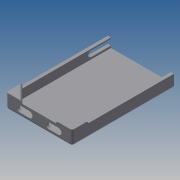
# Autodesk Inventor part: Attempt 3
Saved by Autodesk Inventor 2014 (Build 180170000, 170)
## iProperties
Created: 2014-04-30
Part Number: Attempt 3
Material: Generic
Document SubType Name: Modeling
Designer: 1770749
Density: 1 g/cm^3
Appearance: Default
Author: 1770749
Autodesk Inventor part; units mm, degrees
ref_plane "YZ Plane" through (0, 0, 0) normal (1, 0, 0) x (0, 1, 0)
ref_plane "XZ Plane" through (0, 0, 0) normal (0, 1, 0) x (-1, 0, 0)
ref_plane "XY Plane" through (0, 0, 0) normal (0, 0, 1) x (1, 0, 0)
sketch "Sketch1" plane through (0, 0, 0) normal (0, 0, 1) x (1, 0, 0)
  line L0 (0, 0) -> (59.18, 0)
  line L1 (59.18, 0) -> (59.18, 124.44)
  line L2 (59.18, 124.44) -> (0, 124.44)
  line L3 (0, 124.44) -> (0, 0)
  dimension "d0" = 59.18
  dimension "d1" = 124.44
  constraints: 8 end point, 2 parallel, 1 horizontal, 1 perpendicular
  measures "d0" distance of L2.end L1.end
  measures "d1" distance of L1.end L0.end
sketch "Sketch2" plane through (0, 0, 0) normal (0, 0, 1) x (1, 0, 0)
  line L0 (-3, 127.44) -> (62.18, 127.44)
  line L1 (62.18, 127.44) -> (62.18, -3)
  line L2 (62.18, -3) -> (-3, -3)
  line L3 (-3, -3) -> (-3, 127.44)
  line L4 (59.18, 0) -> (59.18, 124.44) projected
  line L5 (59.18, 124.44) -> (0, 124.44) projected
  line L6 (0, 124.44) -> (0, 0) projected
  line L7 (0, 0) -> (59.18, 0) projected
  dimension "d2" = 3
  dimension "d3" = 3
  dimension "d4" = 3
  dimension "d5" = 3
  constraints: 8 end point, 2 parallel, 1 horizontal, 1 perpendicular
  measures "d2" distance between parallel lines of L1 L4
  measures "d3" distance between parallel lines of L0 L5
  measures "d4" distance between parallel lines of L6 L3
  measures "d5" distance between parallel lines of L2 L7
extrude "Main Extrusion" add sketch "Sketch2" against normal blind 12 contours L0 L1 L2 L3 | L7 L6 L5 L4
extrude "Space for phone" cut sketch "Sketch1" against normal blind 8.97
fillet "Top right corner" radius 2 1 edges at (62.18, 127.44, -6)
fillet "Top left corver" radius 2 1 edges at (-3, 127.44, -6)
fillet "Botton corners" radius 2 2 edges at (62.18, -3, -6) (-3, -3, -6)
fillet "Fillet4" radius 2 8 edges at (61.5942, -2.4142, -12) (29.59, -3, -12) (-2.4142, -2.4142, -12) (-3, 62.22, -12) (-2.4142, 126.8542, -12) (29.59, 127.44, -12) (61.5942, 126.8542, -12) (62.18, 62.22, -12)
sketch "Sketch5" plane through (0, 0, 0) normal (0, 0, 1) x (1, 0, 0)
  arc A0 (-3, -1) -> (-1, -3) centre (-1, -1) ccw projected
  line L0 (60.18, -3) -> (-1, -3) projected
  line L1 (-3, -1) -> (-3, 125.44) projected
  line L2 (-3, 13) -> (13, -3)
  line L3 (-3, 13) -> (19.6274, 13) construction
  line L4 (13, -3) -> (-1, -3)
  line L5 (-3, 13) -> (-3, -1)
  arc A1 (-3, -1) -> (-1, -3) centre (-1, -1) ccw
  line L6 (-1, 127.44) -> (60.18, 127.44) projected
  arc A2 (-1, 127.44) -> (-3, 125.44) centre (-1, 125.44) ccw projected
  line L7 (-3, 111.44) -> (13, 127.44)
  line L8 (-3, 125.44) -> (-3, 111.44)
  line L9 (-1, 127.44) -> (13, 127.44)
  arc A3 (-1, 127.44) -> (-3, 125.44) centre (-1, 125.44) ccw
  line L10 (62.18, 125.44) -> (62.18, -1) projected
  arc A4 (62.18, 125.44) -> (60.18, 127.44) centre (60.18, 125.44) ccw projected
  arc A5 (60.18, -3) -> (62.18, -1) centre (60.18, -1) ccw projected
  line L11 (46.18, 127.44) -> (62.18, 111.44)
  line L12 (46.18, 127.44) -> (60.18, 127.44)
  line L13 (62.18, 125.44) -> (62.18, 111.44)
  arc A6 (62.18, 125.44) -> (60.18, 127.44) centre (60.18, 125.44) ccw
  line L14 (60.18, -3) -> (46.18, -3)
  line L15 (62.18, -1) -> (62.18, 13)
  line L16 (62.18, 13) -> (46.18, -3)
  arc A7 (60.18, -3) -> (62.18, -1) centre (60.18, -1) ccw
  dimension "d18" = 45
  dimension "d21" = 16
  dimension "d22" = 16
  dimension "d23" = 45
  dimension "d26" = 16
  dimension "d27" = 45
  dimension "d28" = 16
  dimension "d29" = 45
  constraints: 26 end point, 10 point on circle, 10 tangent, 8 point on line, 4 centre point, 4 collinear, 3 perpendicular, 1 concentric, 1 equal length, 1 horizontal
  measures "d18" angle of L2 L3
  measures "d21" distance from line of L0 L2.start
  measures "d22" distance from line of L7.start L6
  measures "d23" angle of L1 L7
  measures "d26" distance from line of L6 L11.end
  measures "d27" angle of L10 L11
  measures "d28" distance from line of L14 L15.end
  measures "d29" angle of L10 L16
extrude "Tabs that hold the phone in" add sketch "Sketch5" along normal blind 2 contours L1 L2 L0 A0 | L1 A2 L6 L7 | L16 L10 A5 L0 | L6 A4 L10 L11
sketch "Sketch6" plane through (-1, -3, -10) normal (0, -1, 0) x (1, 0, 0)
  line L0 (61.18, 0) -> (0, 0) projected
  line L1 (61.18, 0) -> (61.18, 12) projected
  line L2 (49.68, 4.37) -> (40.2, 4.37) construction
  line L3 (49.68, 1.37) -> (40.2, 1.37)
  line L4 (40.2, 7.37) -> (49.68, 7.37)
  arc A0 (49.68, 1.37) -> (49.68, 7.37) centre (49.68, 4.37) ccw
  arc A1 (40.2, 7.37) -> (40.2, 1.37) centre (40.2, 4.37) ccw
  point P0 (1, 10)
  point P1 (44.94, 4.37)
  dimension "d33" = 1.37
  dimension "d35" = 3
  dimension "d36" = 9.48
  dimension "d37" = 8.5
  constraints: 8 end point, 4 point on circle, 4 tangent, 2 centre point, 2 parallel, 1 midpoint
  measures "d33" distance between parallel lines of L0 L3
  measures "d35" distance between parallel lines of L2 L4
  measures "d36" distance of L2.start L2.end
  measures "d37" distance edge to line of A0 L1
extrude "Speaker holes" cut sketch "Sketch6" against normal up to next
sketch "Sketch7" plane through (-1, -3, -10) normal (0, -1, 0) x (1, 0, 0)
  line L0 (49.68, 1.37) -> (40.2, 1.37) projected
  line L1 (61.18, 0) -> (0, 0) projected
  line L2 (0, 0) -> (0, 12) projected
  line L3 (20.98, 4.37) -> (11.5, 4.37) construction
  line L4 (20.98, 1.37) -> (11.5, 1.37)
  line L5 (11.5, 7.37) -> (20.98, 7.37)
  arc A0 (20.98, 1.37) -> (20.98, 7.37) centre (20.98, 4.37) ccw
  arc A1 (11.5, 7.37) -> (11.5, 1.37) centre (11.5, 4.37) ccw
  point P0 (1, 10)
  point P1 (16.24, 4.37)
  dimension "d40" = 1.37
  dimension "d41" = 9.48
  dimension "d42" = 8.5
  dimension "d43" = 3
  constraints: 8 end point, 4 point on circle, 4 tangent, 2 centre point, 2 parallel, 1 midpoint
  measures "d40" distance between parallel lines of L1 L4
  measures "d41" distance of L4.start L4.end
  measures "d42" distance edge to line of A1 L2
  measures "d43" distance between parallel lines of L3 L5
extrude "Extrusion8" cut sketch "Sketch7" against normal up to next
fillet "Fillet5" radius 2 4 edges at (5, 119.44, 2) (54.18, 119.44, 2) (5, 5, 2) (54.18, 5, 2)
sketch "Sketch9" plane through (0, 0, -12) normal (0, 0, -1) x (-1, 0, 0)
  line L0 (1, -1) -> (-60.18, -1) projected
  line L1 (-60.18, 125.44) -> (1, 125.44) projected
  line L2 (-60.18, -1) -> (-60.18, 125.44) projected
  line L3 (-50.59, 117.78) -> (-41.14, 117.78) construction
  line L4 (-50.59, 111.78) -> (-41.14, 111.78)
  line L5 (-41.14, 123.78) -> (-50.59, 123.78)
  arc A0 (-50.59, 123.78) -> (-50.59, 111.78) centre (-50.59, 117.78) ccw
  arc A1 (-41.14, 111.78) -> (-41.14, 123.78) centre (-41.14, 117.78) ccw
  point P0 (0, 0)
  point P1 (-45.865, 117.78)
  dimension "d49" = 7.66
  dimension "d50" = 9.59
  dimension "d51" = 19.04
  dimension "d52" = 12
  constraints: 8 end point, 4 point on circle, 4 tangent, 2 centre point, 2 parallel, 1 midpoint
  measures "d49" distance from line of L1 L3.start
  measures "d50" distance from line of L2 L3.start
  measures "d51" distance from line of L3.end L2
  measures "d52" diameter of A1
extrude "Extrusion10" cut sketch "Sketch9" against normal up to next
sketch "Sketch10" plane through (-3, -1, -10) normal (-1, 0, 0) x (0, 0, 1)
  line L0 (10, 14) -> (10, 112.44) projected
  line L1 (10, 125.44) -> (1.03, 125.44) projected
  line L2 (10, 125.44) -> (1.03, 125.44) projected
  line L3 (10, 125.44) -> (1.03, 125.44) projected
  line L4 (1.03, 1) -> (1.03, 125.44) projected
  line L5 (5.91, 108.13) -> (5.91, 79) construction
  line L6 (3.0058, 108.13) -> (3.0058, 79)
  line L7 (8.8142, 79) -> (8.8142, 108.13)
  arc A0 (8.8142, 108.13) -> (3.0058, 108.13) centre (5.91, 108.13) ccw
  arc A1 (3.0058, 79) -> (8.8142, 79) centre (5.91, 79) ccw
  point P0 (10, 1)
  point P1 (5.91, 93.565)
  dimension "d55" = 4.88
  dimension "d56" = 17.31
  dimension "d57" = 46.44
  constraints: 8 end point, 4 point on circle, 4 tangent, 2 centre point, 2 parallel, 1 midpoint
  measures "d55" distance from line of L4 L5.start
  measures "d56" distance from line of L1 L5.start
  measures "d57" distance from line of L1 L5.end
extrude "Extrusion11" cut sketch "Sketch10" against normal up to next
sketch "Sketch11" plane through (-1, 127.44, -10) normal (0, 1, 0) x (1, 0, 0)
  line L0 (61.18, -12) -> (50.0084, -12) projected
  line L1 (0, 0) -> (61.18, 0) projected
  line L2 (11, -10) -> (50.18, -10) projected
  line L3 (60.18, -10) -> (60.18, -1.03) projected
  line L4 (1, -1.03) -> (60.18, -1.03) projected
  line L5 (40.54, -4.77) -> (50.12, -4.77) construction
  line L6 (40.54, -7.6395) -> (50.12, -7.6395)
  line L7 (50.12, -1.9005) -> (40.54, -1.9005)
  arc A0 (40.54, -1.9005) -> (40.54, -7.6395) centre (40.54, -4.77) ccw
  arc A1 (50.12, -7.6395) -> (50.12, -1.9005) centre (50.12, -4.77) ccw
  point P0 (1, -10)
  point P1 (45.33, -4.77)
  dimension "d60" = 3.74
  dimension "d61" = 10.06
  dimension "d62" = 9.58
  constraints: 8 end point, 4 point on circle, 4 tangent, 2 centre point, 2 parallel, 1 midpoint
  measures "d60" distance from line of L4 L5.end
  measures "d61" distance from line of L3 L5.end
  measures "d62" distance of L5.end L5.start
extrude "Extrusion12" cut sketch "Sketch11" against normal up to next
ref_plane "Work Plane1" through (-1, 97.44, -10) normal (0, 1, 0) x (1, 0, 0)
split body "Split1" result two bodies by plane through (-1, 97.44, -10) normal (0, 1, 0) first body at (11.0612, 113.3123, -11.5)
sketch "Sketch12" plane through (-1, 97.44, -12) normal (0, -1, 0) x (1, 0, 0)
  line L0 (60.18, 3.03) -> (1, 3.03) projected
  circle A0 centre (-0.5, 3.5029) radius 0.75
  circle A1 centre (61.68, 3.5029) radius 0.75
  circle A2 centre (61.68, 10.0883) radius 0.75
  line L1 (58.4184, 1.53) -> (2.785, 1.53) construction
  line L2 (58.4184, 2.28) -> (2.785, 2.28)
  line L3 (2.785, 0.78) -> (58.4184, 0.78)
  arc A3 (58.4184, 0.78) -> (58.4184, 2.28) centre (58.4184, 1.53) ccw
  arc A4 (2.785, 2.28) -> (2.785, 0.78) centre (2.785, 1.53) ccw
  point P0 (1, 12)
  point P1 (30.6017, 1.53)
  dimension "d66" = 1.5
  dimension "d67" = 1.5
  dimension "d68" = 1.5
  dimension "d69" = 0.75
  constraints: 8 end point, 5 centre point, 4 point on circle, 4 tangent, 2 parallel, 1 midpoint
  measures "d66" diameter of A0
  measures "d67" diameter of A2
  measures "d68" diameter of A4
  measures "d69" distance between parallel lines of L2 L0
extrude "Extrusion13" add sketch "Sketch12" along normal blind 10 bodies 2
sketch "Sketch13" plane through (-1, 97.44, -12) normal (0, 1, 0) x (1, 0, 0)
  circle A0 centre (-0.5, -3.5029) radius 0.75 projected
  circle A1 centre (61.68, -3.5029) radius 0.75 projected
  circle A2 centre (61.68, -10.0883) radius 0.75 projected
  line L0 (58.4184, -2.28) -> (2.785, -2.28) projected
  arc A3 (2.785, -0.78) -> (2.785, -2.28) centre (2.785, -1.53) ccw projected
  line L1 (2.785, -0.78) -> (58.4184, -0.78) projected
  arc A4 (58.4184, -2.28) -> (58.4184, -0.78) centre (58.4184, -1.53) ccw projected
  circle A5 centre (61.68, -10.0883) radius 0.75 projected
  circle A6 centre (61.68, -10.0883) radius 0.75
  circle A7 centre (61.68, -3.5029) radius 0.75
  circle A8 centre (-0.5, -3.5029) radius 0.75
  line L2 (58.4184, -1.53) -> (2.785, -1.53) construction
  line L3 (58.4184, -0.78) -> (2.785, -0.78)
  line L4 (2.785, -2.28) -> (58.4184, -2.28)
  arc A9 (58.4184, -2.28) -> (58.4184, -0.78) centre (58.4184, -1.53) ccw
  arc A10 (2.785, -0.78) -> (2.785, -2.28) centre (2.785, -1.53) ccw
  point P0 (1, -12)
  point P1 (30.6017, -1.53)
  constraints: 8 end point, 5 centre point, 4 point on circle, 4 tangent, 3 coincident, 2 concentric, 2 parallel, 1 midpoint
extrude "Extrusion14" cut sketch "Sketch13" against normal blind 10 bodies 3
